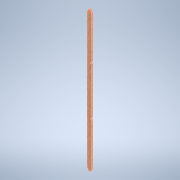
# Autodesk Inventor part: ReedRail_V2
Saved by Autodesk Inventor 2022.2 (Build 262287000, 287)
## iProperties
Created: 2023-03-06
Part Number: ReedRail_V2
Material: Wood (Oak)
Document SubType Name: Modeling
Designer: jaege
Density: 0.76 g/cm^3
Appearance: Red Oak - Natural Low Gloss
Author: jaege
Autodesk Inventor part; units mm, degrees
ref_plane "YZ Plane" through (0, 0, 0) normal (1, 0, 0) x (0, 1, 0)
ref_plane "XZ Plane" through (0, 0, 0) normal (0, 1, 0) x (-1, 0, 0)
ref_plane "XY Plane" through (0, 0, 0) normal (0, 0, 1) x (1, 0, 0)
sketch "Sketch1" plane through (0, 0, 0) normal (0, 0, 1) x (1, 0, 0)
  line L0 (-5, 173) -> (-3, 173)
  line L1 (5, 173) -> (5, -173)
  line L2 (5, -173) -> (3, -173)
  line L3 (-5, -173) -> (-5, 173)
  circle A0 centre (5, 62.5) radius 2.5
  circle A1 centre (5, -61) radius 2.5
  line L4 (-3, 173) -> (3, 173) construction
  line L5 (3, 173) -> (3, 177)
  line L6 (3, 177) -> (-3, 177)
  line L7 (-3, 177) -> (-3, 173)
  line L8 (-3, -173) -> (3, -173) construction
  line L9 (3, -173) -> (3, -177)
  line L10 (3, -177) -> (-3, -177)
  line L11 (-3, -177) -> (-3, -173)
  line L12 (0, 173) -> (0, -173)
  line L13 (-3, 173) -> (3, 173) construction
  line L14 (3, 173) -> (5, 173)
  line L15 (-3, -173) -> (-5, -173)
  line L16 (3, -173) -> (-3, -173) construction
  point P0 (0, 0)
  point P1 (0, 0)
  point P2 (5, -63.5)
  point P3 (5, -58.5)
  point P4 (5, 60)
  point P5 (5, 65)
  dimension "d0" = 5
  dimension "d4" = 10
  dimension "d5" = 6
  dimension "d6" = 4
  dimension "d7" = 346
  dimension "d8" = 110.5
  dimension "d9" = 112
  constraints: 34 end point, 14 parallel, 5 horizontal, 5 perpendicular, 4 point on line, 3 midpoint, 2 centre point, 1 coincident, 1 collinear, 1 equal radius, 1 other
  measures "d0" diameter of A0
  measures "d4" distance between parallel lines of L1 L3
  measures "d5" distance between parallel lines of L5 L7
  measures "d6" distance of L10.end L8.start
  measures "d7" distance of L3.start L0.start
  measures "d8" distance of A0.centre L1.start
  measures "d9" distance of L1.end A1.centre
extrude "Extrusion1" add sketch "Sketch1" along normal blind 4 contours L0 L7 L6 L5 L14 L1 A0 A1 L2 L9 L10 L11 L15 L3
body "Solid1"
